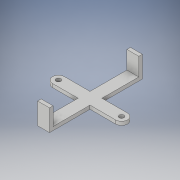
# Autodesk Inventor part: Battery Restraint
Saved by Autodesk Inventor 2019 (Build 230136000, 136)
## iProperties
Created: 2018-11-13
Part Number: Battery Restraint
Material: Generic
Document SubType Name: Modeling
Designer: Billy
Density: 1 g/cm^3
Appearance: Default
Author: Billy
Autodesk Inventor part; units mm, degrees
ref_plane "YZ Plane" through (0, 0, 0) normal (1, 0, 0) x (0, 1, 0)
ref_plane "XZ Plane" through (0, 0, 0) normal (0, 1, 0) x (-1, 0, 0)
ref_plane "XY Plane" through (0, 0, 0) normal (0, 0, 1) x (1, 0, 0)
sketch "Sketch1" plane through (0, 0, 0) normal (0, 1, 0) x (-1, 0, 0)
  circle A0 centre (0, 0) radius 2
  circle A1 centre (53, 0) radius 2
  arc A2 (53, -5) -> (53, 5) centre (53, 0) ccw
  arc A3 (0, 5) -> (0, -5) centre (0, 0) ccw
  line L0 (31.5, 37.5) -> (31.5, 5)
  line L1 (31.5, -5) -> (31.5, -39)
  line L2 (21.5, 37.5) -> (21.5, 5)
  line L3 (21.5, -5) -> (21.5, -39)
  line L4 (31.5, 39) -> (21.5, 39)
  line L5 (21.5, 39) -> (21.5, 36)
  line L6 (31.5, 36) -> (31.5, 39)
  line L7 (31.5, -39) -> (21.5, -39)
  line L8 (53, 5) -> (31.5, 5)
  line L9 (21.5, 5) -> (0, 5)
  line L10 (53, -5) -> (31.5, -5)
  line L11 (21.5, -5) -> (0, -5)
  dimension "d0" = 4
  dimension "d1" = 4
  dimension "d2" = 10
  dimension "d3" = 10
  dimension "d8" = 3
  constraints: 24 end point, 5 parallel, 4 centre point, 4 point on circle, 4 tangent, 3 coincident, 3 horizontal, 2 midpoint, 2 point on line, 1 perpendicular
  measures "d0" diameter of A0
  measures "d1" diameter of A1
  measures "d2" diameter of A2
  measures "d3" diameter of A3
  measures "d8" distance of L5.end L4.end
extrude "Extrusion1" add sketch "Sketch1" along normal blind 3
sketch "Sketch2" plane through (0, 3, 0) normal (0, 1, 0) x (1, 0, 0)
  circle A0 centre (-53, 0) radius 2 projected
  circle A1 centre (0, 0) radius 2 projected
  line L0 (-53, -5) -> (-31.5, -5) projected
  line L1 (-31.5, -5) -> (-31.5, -39) projected
  line L2 (-31.5, -39) -> (-21.5, -39) projected
  line L3 (-21.5, -39) -> (-21.5, -5) projected
  line L4 (-21.5, -5) -> (0, -5) projected
  arc A2 (0, -5) -> (0, 5) centre (0, 0) ccw projected
  line L5 (0, 5) -> (-21.5, 5) projected
  line L6 (-21.5, 5) -> (-21.5, 39) projected
  line L7 (-21.5, 39) -> (-31.5, 39) projected
  line L8 (-31.5, 39) -> (-31.5, 5) projected
  line L9 (-31.5, 5) -> (-53, 5) projected
  arc A3 (-53, 5) -> (-53, -5) centre (-53, 0) ccw projected
  line L10 (-21.5, 5) -> (-21.5, 39) projected
  line L11 (-31.5, 39) -> (-21.5, 39)
  line L12 (-21.5, 39) -> (-21.5, 36)
  line L13 (-21.5, 36) -> (-31.5, 36)
  line L14 (-31.5, 36) -> (-31.5, 39)
  line L15 (-21.5, -39) -> (-21.5, -5) projected
  line L16 (-31.5, -39) -> (-21.5, -39)
  line L17 (-21.5, -39) -> (-21.5, -36)
  line L18 (-21.5, -36) -> (-31.5, -36)
  line L19 (-31.5, -36) -> (-31.5, -39)
  dimension "d11" = 3
  dimension "d12" = 3
  constraints: 16 end point, 4 parallel, 2 horizontal, 2 perpendicular, 2 point on line
  measures "d11" distance of L11.end L12.end
  measures "d12" distance of L17.end L16.end
extrude "Extrusion2" add sketch "Sketch2" along normal blind 15 contours L18 L3 L2 L1 | L8 L7 L6 L13
body "Solid1"
